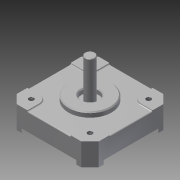
# Autodesk Inventor part: stepper_front
Saved by Autodesk Inventor 2013 (Build 170138000, 138)
## iProperties
Shininess: 50.0
Created: 2011-05-14
Part Number: stepper_front
Document SubType Name: Modeling
Designer: Noa Izumi
Material: Default
Density: 1 g/cm^3
Density: 0.0
Volumn: 0.0
Area: 0.0
PropertySet Name: Model Information
Control State: 0
Master: False
Checked Out: False
Author: Noa Izumi
Autodesk Inventor part; units mm, degrees
ref_plane "YZ Plane" through (0, 0, 0) normal (1, 0, 0) x (0, 1, 0)
ref_plane "XZ Plane" through (0, 0, 0) normal (0, 1, 0) x (-1, 0, 0)
ref_plane "XY Plane" through (0, 0, 0) normal (0, 0, 1) x (1, 0, 0)
sketch "Sketch1" plane through (0, 0, 0) normal (0, 0, 1) x (1, 0, 0)
  line L0 (0, 0) -> (42, 0)
  line L1 (42, 0) -> (42, 42)
  line L2 (42, 42) -> (0, 42)
  line L3 (0, 42) -> (0, 0)
  dimension "d0" = 42
  dimension "d1" = 42
  constraints: 8 end point, 2 parallel, 1 horizontal, 1 perpendicular
  measures "d0" distance of L2.end L0.start
  measures "d1" distance of L0.start L0.end
extrude "Extrusion1" add sketch "Sketch1" along normal blind 11.5
chamfer "Chamfer1" distance 4.5 angle 45 4 edges at (0, 0, 5.75) (42, 0, 5.75) (42, 42, 5.75) (0, 42, 5.75)
sketch "Sketch2" plane through (0, 0, 11.5) normal (0, 0, 1) x (1, 0, 0)
  line L0 (4.5, 42) -> (37.5, 42) projected
  line L1 (0, 4.5) -> (0, 37.5) projected
  line L2 (37.5, 0) -> (4.5, 0) projected
  line L3 (42, 37.5) -> (42, 4.5) projected
  line L4 (10, 0) -> (10, 6)
  line L5 (10, 36) -> (10, 42)
  line L6 (0, 32) -> (6, 32)
  line L7 (36, 32) -> (42, 32)
  line L8 (0, 10) -> (6, 10)
  line L9 (36, 10) -> (42, 10)
  line L10 (32, 42) -> (32, 36)
  line L11 (32, 6) -> (32, 0)
  arc A0 (6, 32) -> (10, 36) centre (6, 36) ccw
  arc A1 (32, 36) -> (36, 32) centre (36, 36) ccw
  arc A2 (36, 10) -> (32, 6) centre (36, 6) ccw
  arc A3 (10, 6) -> (6, 10) centre (6, 6) ccw
  dimension "d10" = 4
  constraints: 16 end point, 10 parallel, 8 point on circle, 8 point on line, 8 tangent, 4 centre point, 4 perpendicular, 3 equal radius
  measures "d10" radius of A0
extrude "Extrusion2" cut sketch "Sketch2" against normal blind 0.5
fillet "Fillet1" radius 0.5 12 edges at (8.8284, 8.8284, 11) (10, 3, 11) (3, 10, 11) (3, 32, 11) (8.8284, 33.1716, 11) (10, 39, 11) (33.1716, 33.1716, 11) (32, 39, 11) (39, 32, 11) (39, 10, 11) (33.1716, 8.8284, 11) (32, 3, 11)
fillet "Fillet2" radius 0.5 12 edges at (0, 21, 11) (0, 10.1463, 11.1463) (0, 31.8537, 11.1463) (21, 42, 11) (10.1463, 42, 11.1463) (31.8537, 42, 11.1463) (42, 21, 11) (42, 31.8537, 11.1463) (42, 10.1463, 11.1463) (21, 0, 11) (31.8537, 0, 11.1463) (10.1463, 0, 11.1463)
sketch "Sketch3" plane through (0, 0, 11) normal (0, 0, 1) x (1, 0, 0)
  circle A0 centre (21, 21) radius 11
  line L0 (10.5, 0) -> (31.5, 0) projected
  line L1 (0, 31.5) -> (0, 10.5) projected
  circle A1 centre (21, 21) radius 4.5
  dimension "d15" = 22
  dimension "d16" = 21
  dimension "d17" = 21
  dimension "d18" = 9
  constraints: 2 centre point, 1 coincident
  measures "d15" diameter of A0
  measures "d16" distance from line of L0 A0.centre
  measures "d17" distance from line of L1 A0.centre
  measures "d18" diameter of A1
extrude "Extrusion3" add sketch "Sketch3" along normal blind 2.5
chamfer "Chamfer2" distance 0.5 angle 45 2 edges at (10, 21, 13.5) (16.5, 21, 13.5)
sketch "Sketch4" plane through (21, 21, 11) normal (0, 0, 1) x (1, 0, 0)
  circle A0 centre (0, 0) radius 4.5 projected
  circle A1 centre (0, 0) radius 2.5
  dimension "d23" = 5
  constraints: 1 centre point, 1 coincident
  measures "d23" diameter of A1
extrude "Extrusion4" add sketch "Sketch4" along normal blind 20 contours A1
sketch "Sketch5" plane through (0, 0, 11.5) normal (0, 0, 1) x (1, 0, 0)
  arc A0 (10, 6) -> (6, 10) centre (6, 6) ccw projected
  point P0 (36, 6)
  point P1 (6, 36)
  point P2 (36, 36)
  dimension "d28" = 30
  dimension "d29" = 30
  constraints: 1 coincident
  measures "d28" distance of point (36, 6) A0.centre
  measures "d29" distance of A0.centre point (6, 36)
hole "Hole1" at (6, 6, 11.5) at (36, 6, 11.5) at (6, 36, 11.5) at (36, 36, 11.5) direction (0, 0, -1) diameter 2.459 end through all thread size "M3x0.5" class "6H" standard "ANSI Metric M Profile"
sketch "Sketch6" plane through (0, 0, 0) normal (0, 0, -1) x (-1, 0, 0)
  line L0 (-42, 4.5) -> (-42, 37.5) projected
  line L1 (-4.5, 0) -> (-37.5, 0) projected
  circle A0 centre (-21, 21) radius 25.25
  dimension "d37" = 50.5
  dimension "d38" = 21
  dimension "d39" = 21
  constraints: 1 centre point
  measures "d37" diameter of A0
  measures "d38" distance from line of L0 A0.centre
  measures "d39" distance from line of L1 A0.centre
extrude "Extrusion5" cut sketch "Sketch6" against normal blind 2
chamfer "倒角4" distance 0.25 angle 45 1 edges at (18.5, 21, 31)
